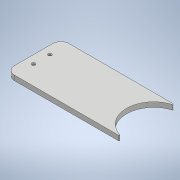
# Autodesk Inventor part: Поршень
Saved by Autodesk Inventor 2020 (Build 240168000, 168)
## iProperties
Created: 2019-12-26
Part Number: Поршень
Material: Типовые
Document SubType Name: Modeling
Designer: Css38
Density: 1 g/cm^3
Appearance: По умолчанию
Author: Css38
Autodesk Inventor part; units mm, degrees
ref_plane "YZ Plane" through (0, 0, 0) normal (1, 0, 0) x (0, 1, 0)
ref_plane "XZ Plane" through (0, 0, 0) normal (0, 1, 0) x (-1, 0, 0)
ref_plane "XY Plane" through (0, 0, 0) normal (0, 0, 1) x (1, 0, 0)
sketch "Эскиз1" plane through (0, 0, 0) normal (0, 0, 1) x (1, 0, 0)
  line L0 (51.75, 11.75) -> (0, 11.75)
  line L1 (0, -11.75) -> (51.75, -11.75)
  arc A0 (51.75, 11.75) -> (51.75, -11.75) centre (51.75, 0) ccw
  line L2 (0, -11.75) -> (0, 11.75)
  line L3 (0, 0) -> (40, 0) construction
  line L4 (0, 0) -> (0, 11.75) construction
  line L5 (0, 11.75) -> (0, 11.25)
  point P0 (20, 0)
  dimension "d0" = 11.75
  dimension "d47" = 40
  constraints: 12 end point, 5 point on circle, 3 midpoint, 2 coincident, 2 collinear, 2 horizontal, 2 parallel, 2 point on line, 2 tangent, 1 centre point, 1 horizontal alignment, 1 vertical alignment
  measures "d0" radius of A0
  measures "d47" distance of L3.start L3.end
extrude "Выдавливание3" add sketch "Эскиз1" along normal blind 2.1
fillet "Сопряжение3" radius 0.25 2 edges at (51.75, 11.75, 1.05) (51.75, -11.75, 1.05)
fillet "Сопряжение4" radius 3.5 2 edges at (0, -11.75, 1.05) (0, 11.75, 1.05)
sketch "Эскиз6" plane through (0, 0, 2.1) normal (0, 0, 1) x (1, 0, 0)
  arc A0 (48.3936, 11.2604) -> (48.3936, -11.2604) centre (51.75, 0) ccw construction
  line L0 (40, 0) -> (0, 0) construction
  line L1 (0, -11.75) -> (0, 11.75) construction
  circle A1 centre (3.5, 3.5) radius 0.5
  line L2 (3.5, 3.5) -> (0, 3.5) construction
  line L3 (3.5, 3.5) -> (3.5, 0) construction
  circle A2 centre (3.5, -3.5) radius 0.5
  point P0 (48.3222, -11.75)
  dimension "d58" = 1
  dimension "d59" = 3.5
  constraints: 6 end point, 3 perpendicular, 2 centre point, 2 point on line, 1 midpoint, 1 point on circle, 1 symmetric about line, 1 other
  measures "d58" diameter of A1
  measures "d59" distance of L2.start L2.end
hole "Отверстие1" at (3.5, -3.5, 2.1) at (3.5, 3.5, 2.1) direction (0, 0, -1) diameter 1 end through all countersink diameter 1.5 countersink angle 90
